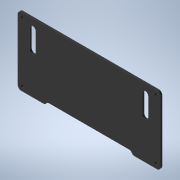
# Autodesk Inventor part: CONTROLBOARD_KLEP
Saved by Autodesk Inventor 2020 (Build 240168000, 168)
## iProperties
Created: 2020-06-09
Part Number: CONTROLBOARD_KLEP
Material: Generic
Document SubType Name: Modeling
Designer: Gebruiker
Density: 1 g/cm^3
Appearance: Default
Author: Gebruiker
Autodesk Inventor part; units mm, degrees
ref_plane "YZ Plane" through (0, 0, 0) normal (1, 0, 0) x (0, 1, 0)
ref_plane "XZ Plane" through (0, 0, 0) normal (0, 1, 0) x (-1, 0, 0)
ref_plane "XY Plane" through (0, 0, 0) normal (0, 0, 1) x (1, 0, 0)
sketch "Sketch1" plane through (0, 0, 0) normal (0, 0, 1) x (1, 0, 0)
  line L0 (-92.5, -50) -> (92.5, -50)
  line L1 (92.5, -50) -> (92.5, 50)
  line L2 (92.5, 50) -> (-92.5, 50)
  line L3 (-92.5, 50) -> (-92.5, -50)
  line L4 (-92.5, -50) -> (92.5, 50) construction
  line L5 (92.5, -50) -> (-92.5, 50) construction
  line L6 (70, 55) -> (115, 55)
  line L7 (115, 55) -> (115, 45)
  line L8 (115, 45) -> (70, 45)
  line L9 (70, 45) -> (70, 55)
  line L10 (70, 55) -> (115, 45) construction
  line L11 (115, 55) -> (70, 45) construction
  line L12 (70, -45) -> (115, -45)
  line L13 (115, -45) -> (115, -55)
  line L14 (115, -55) -> (70, -55)
  line L15 (70, -55) -> (70, -45)
  line L16 (70, -45) -> (115, -55) construction
  line L17 (115, -45) -> (70, -55) construction
  line L18 (-115, -45) -> (-70, -45)
  line L19 (-70, -45) -> (-70, -55)
  line L20 (-70, -55) -> (-115, -55)
  line L21 (-115, -55) -> (-115, -45)
  line L22 (-115, -45) -> (-70, -55) construction
  line L23 (-70, -45) -> (-115, -55) construction
  line L24 (-115, 55) -> (-70, 55)
  line L25 (-70, 55) -> (-70, 45)
  line L26 (-70, 45) -> (-115, 45)
  line L27 (-115, 45) -> (-115, 55)
  line L28 (-115, 55) -> (-70, 45) construction
  line L29 (-70, 55) -> (-115, 45) construction
  line L30 (70, 45) -> (115, 45)
  line L31 (115, 45) -> (115, -45)
  line L32 (115, -45) -> (70, -45)
  line L33 (70, -45) -> (70, 45)
  line L34 (70, 45) -> (115, -45) construction
  line L35 (115, 45) -> (70, -45) construction
  line L36 (-115, 45) -> (-70, 45)
  line L37 (-70, 45) -> (-70, -45)
  line L38 (-70, -45) -> (-115, -45)
  line L39 (-115, -45) -> (-115, 45)
  line L40 (-115, 45) -> (-70, -45) construction
  line L41 (-70, 45) -> (-115, -45) construction
  line L42 (115, 45) -> (115, 25)
  line L43 (115, -45) -> (115, -25)
  line L44 (-115, -45) -> (-115, -25)
  line L45 (-115, 45) -> (-115, 25)
  line L46 (70, 55) -> (-70, 55)
  line L47 (-70, 55) -> (-70, 50)
  line L48 (-70, 50) -> (70, 50)
  line L49 (70, 50) -> (70, 55)
  point P0 (0, 0)
  point P1 (0, 0)
  point P2 (92.5, 0)
  point P3 (-92.5, 0)
  point P4 (-70, -50)
  point P5 (70, -50)
  dimension "d0" = 185
  dimension "d1" = 100
  dimension "d2" = 45
  dimension "d3" = 10
  dimension "d4" = 45
  dimension "d5" = 10
  dimension "d6" = 45
  dimension "d7" = 45
  dimension "d8" = 10
  dimension "d9" = 45
  dimension "d10" = 90
  dimension "d11" = 20
  dimension "d12" = 20
  dimension "d13" = 20
  dimension "d14" = 20
  dimension "d15" = 45
  constraints: 100 end point, 17 midpoint, 16 parallel, 8 horizontal, 8 perpendicular, 6 point on line, 1 collinear
  measures "d0" distance of L2.end L1.end
  measures "d1" distance of L1.end L1.start
  measures "d2" distance of L8.start L8.end
  measures "d3" distance of L7.start L8.start
  measures "d4" distance of L14.start L14.end
  measures "d5" distance of L43.start L14.start
  measures "d6" distance of L19.end L20.end
  measures "d7" distance of L26.start L45.start
  measures "d8" distance of L24.end L26.start
  measures "d9" distance of L31.end L33.start
  measures "d10" distance of L37.start L37.end
  measures "d11" distance of L8.start L42.end
  measures "d12" distance of L43.start L43.end
  measures "d13" distance of L44.start L44.end
  measures "d14" distance of L45.start L45.end
  measures "d15" distance of L37.end L39.start
extrude "Extrusion1" add sketch "Sketch1" against normal blind 3
fillet "Fillet1" radius 5 8 edges at (-115, 55, -1.5) (115, 55, -1.5) (115, -55, -1.5) (70, -55, -1.5) (70, -50, -1.5) (-70, -50, -1.5) (-70, -55, -1.5) (-115, -55, -1.5)
sketch "Sketch2" plane through (0, 0, 0) normal (0, 0, 1) x (1, 0, 0)
  circle A0 centre (-91, 40) radius 5
  circle A1 centre (-91, 10) radius 5
  line L0 (-96, 40) -> (-96, 10)
  line L1 (-86, 10) -> (-86, 40)
  line L2 (-73.6603, 55) -> (-110, 55) projected
  line L3 (-115, 50) -> (-115, -50) projected
  circle A2 centre (-108, 48) radius 2.25
  line L4 (0, 60.4736) -> (0, -65.7733) construction
  circle A3 centre (91, 40) radius 5
  circle A4 centre (91, 10) radius 5
  line L5 (96, 40) -> (96, 10)
  line L6 (86, 10) -> (86, 40)
  circle A5 centre (108, 48) radius 2.25
  line L7 (-147.6516, 0) -> (131.888, 0) construction
  circle A6 centre (-108, -48) radius 2.25
  circle A7 centre (108, -48) radius 2.25
  point P0 (0, 0)
  dimension "d19" = 10
  dimension "d20" = 10
  dimension "d24" = 15
  dimension "d25" = 24
  dimension "d26" = 24
  dimension "d27" = 19
  dimension "d28" = 45
  dimension "d32" = 7
  dimension "d33" = 7
  constraints: 12 end point, 9 symmetric about line, 8 centre point, 8 point on circle, 3 tangent, 1 horizontal, 1 vertical, 5 other
  measures "d19" diameter of A0
  measures "d20" diameter of A1
  measures "d24" distance from line of L2 A0.centre
  measures "d25" distance from line of L3 A0.centre
  measures "d26" distance from line of L3 A1.centre
  measures "d27" distance between parallel lines of L3 L0
  measures "d28" distance from line of L2 A1.centre
  measures "d32" distance from line of L2 A2.centre
  measures "d33" distance from line of L3 A2.centre
extrude "Extrusion2" cut sketch "Sketch2" against normal blind 3
body "Solid1"
